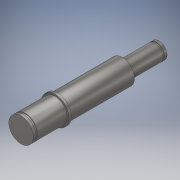
# Autodesk Inventor part: Main Vert Axle
Saved by Autodesk Inventor 2019.4 (Build 234330000, 330)
## iProperties
Created: 2019-11-30
Part Number: Main Vert Axle
Material: Stainless Steel
Document SubType Name: Modeling
Designer: admin
Density: 8 g/cm^3
Appearance: Semi-Polished
Mass: 114.689 g
Surface Area: 44.1694 cm^2
Volume: 14.3361 cm^3
Author: admin
Autodesk Inventor part; units mm, degrees
ref_plane "YZ Plane" through (0, 0, 0) normal (1, 0, 0) x (0, 1, 0)
ref_plane "XZ Plane" through (0, 0, 0) normal (0, 1, 0) x (-1, 0, 0)
ref_plane "XY Plane" through (0, 0, 0) normal (0, 0, 1) x (1, 0, 0)
sketch "Sketch1" plane through (0, 0, 0) normal (1, 0, 0) x (0, 1, 0)
  line L0 (0, 0) -> (7.5, 0)
  line L1 (7.5, -20.8) -> (8.5, -20.8)
  line L2 (8.5, -20.8) -> (8.5, -22.3)
  line L3 (8.5, -22.3) -> (7.5, -22.3)
  line L4 (7.5, 0) -> (7.5, -1.5)
  line L5 (7.5, -1.5) -> (7.15, -1.5)
  line L6 (7.15, -1.5) -> (7.15, -2.6)
  line L7 (7.15, -2.6) -> (7.5, -2.6)
  line L8 (7.5, -2.6) -> (7.5, -20.8)
  line L9 (5, -82.955) -> (5, -84.455)
  line L10 (5, -84.455) -> (0, -84.455)
  line L11 (0, -84.455) -> (0, 0)
  line L12 (7.5, -22.3) -> (7.5, -62)
  line L13 (7.5, -62) -> (5, -62)
  line L14 (5, -62) -> (5, -81.855)
  line L15 (5, -81.855) -> (4.65, -81.855)
  line L16 (4.65, -81.855) -> (4.65, -82.955)
  line L17 (4.65, -82.955) -> (5, -82.955)
  dimension "d0" = 7.5
  dimension "d1" = 8.5
  dimension "d3" = 1.5
  dimension "d4" = 18.2
  dimension "d5" = 1.5
  dimension "d6" = 0.35
  dimension "d7" = 1.1
  dimension "d18" = 5
  dimension "d19" = 7.5
  dimension "d20" = 1.1
  dimension "d21" = 0.35
  dimension "d22" = 59.555
  dimension "d23" = 1.5
  dimension "d24" = 39.7
  constraints: 37 end point, 11 perpendicular, 2 horizontal, 2 vertical, 1 collinear, 1 point on line
  measures "d0" distance between parallel lines of L11 L8
  measures "d1" distance between parallel lines of L11 L2
  measures "d3" distance of L0.end L4.end
  measures "d4" distance of L7.end L1.start
  measures "d5" distance of L1.end L2.end
  measures "d6" distance of L6.end L7.end
  measures "d7" distance of L5.end L6.end
  measures "d18" distance between parallel lines of L11 L14
  measures "d19" distance between parallel lines of L11 L12
  measures "d20" distance of L15.end L16.end
  measures "d21" distance of L14.end L15.end
  measures "d22" distance between parallel lines of L3 L15
  measures "d23" distance of L9.start L9.end
  measures "d24" distance between parallel lines of L3 L13
revolve "Revolution1" add sketch "Sketch1" angle 360 about axis through (0, 0, -84.455) along (0, 0, 1)
body "Solid1"
